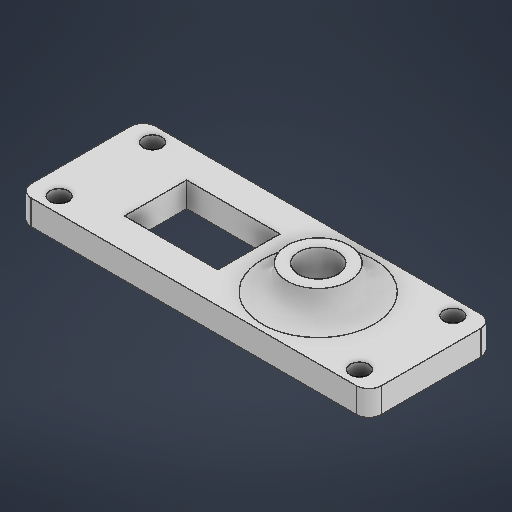
# Autodesk Inventor part: back_servo_support
Saved by Autodesk Inventor 2026.1 (Build 301233000, 233)
## iProperties
Created: 2025-10-30
Part Number: back_servo_support
Material: Generic
Document SubType Name: Modeling
Designer: emanuel
Density: 1 g/cm^3
Appearance: Default
Author: emanuel
Autodesk Inventor part; units mm, degrees
ref_plane "YZ Plane" through (0, 0, 0) normal (1, 0, 0) x (0, 1, 0)
ref_plane "XZ Plane" through (0, 0, 0) normal (0, 1, 0) x (-1, 0, 0)
ref_plane "XY Plane" through (0, 0, 0) normal (0, 0, 1) x (1, 0, 0)
sketch "Sketch1" plane through (0, 0, 0) normal (0, 1, 0) x (-1, 0, 0)
  line L0 (0, 0) -> (48.3, 0)
  line L1 (48.3, 0) -> (48.3, -15)
  line L2 (48.3, -15) -> (0, -15)
  line L3 (0, -15) -> (0, 0)
  circle A0 centre (48.3, 0) radius 1.5
  circle A1 centre (48.3, -15) radius 1.5
  circle A2 centre (0, 0) radius 1.5
  circle A3 centre (0, -15) radius 1.5
  line L4 (48.3, -15) -> (52.3, -15)
  line L5 (52.3, -15) -> (52.3, -17.5)
  line L6 (52.3, -17.5) -> (48.3, -17.5)
  line L7 (48.3, -17.5) -> (48.3, -15)
  line L8 (0, 0) -> (-4, 0)
  line L9 (-4, 0) -> (-4, 2.5)
  line L10 (-4, 2.5) -> (0, 2.5)
  line L11 (0, 2.5) -> (0, 0)
  line L12 (-4, 2.5) -> (52.3, 2.5)
  line L13 (52.3, 2.5) -> (52.3, -17.5)
  line L14 (52.3, -17.5) -> (-4, -17.5)
  line L15 (-4, -17.5) -> (-4, 2.5)
  dimension "d0" = 48.3
  dimension "d1" = 15
  dimension "d2" = 3
  dimension "d3" = 3
  dimension "d4" = 3
  dimension "d5" = 3
  dimension "d6" = 4
  dimension "d7" = 2.5
  dimension "d8" = 4
  dimension "d9" = 2.5
  constraints: 32 end point, 8 parallel, 4 centre point, 4 coincident, 4 horizontal, 4 perpendicular
  measures "d0" distance of L1.end L2.end
  measures "d1" distance of L0.end L1.end
  measures "d2" diameter of A0
  measures "d3" diameter of A1
  measures "d4" diameter of A2
  measures "d5" diameter of A3
  measures "d6" distance of L5.end L6.end
  measures "d7" distance of L4.end L5.end
  measures "d8" distance of L9.end L10.end
  measures "d9" distance of L8.end L9.end
extrude "Extrusion1" add sketch "Sketch1" along normal blind 4 contours A2 L11 L12 L13 L4 A1 L1 A0 L0 | L0 A0 L1 A1 L2 A3 L3 A2 | L3 A3 L2 A1 L7 L14 L15 L8 A2 | L8 L9 L10 L11 A2 | L7 A1 L4 L5 L6
sketch "Sketch2" plane through (0, 4, 0) normal (0, 1, 0) x (1, 0, 0)
  line L0 (4, -2.5) -> (4, 17.5) projected
  line L1 (4, -2.5) -> (-14.15, -2.5)
  line L2 (-14.15, -2.5) -> (-14.15, 7.5)
  line L3 (-14.15, 7.5) -> (4, 7.5)
  line L4 (4, 7.5) -> (4, -2.5)
  circle A0 centre (-14.15, 7.5) radius 5
  circle A1 centre (-14.15, 7.5) radius 3.15
  point P0 (0, 0)
  dimension "d12" = 18.15
  dimension "d13" = 10
  dimension "d14" = 10
  dimension "d19" = 6.3
  constraints: 8 end point, 2 centre point, 2 parallel, 1 coincident, 1 horizontal, 1 perpendicular
  measures "d12" distance of L2.end L3.end
  measures "d13" distance of L1.end L2.end
  measures "d14" diameter of A0
  measures "d19" diameter of A1
extrude "Extrusion2" add sketch "Sketch2" along normal blind 4 contours A0 L2 A1 L3 | L3 A1 L2 A0
extrude "Extrusion3" cut sketch "Sketch2" against normal blind 3 contours A1 L2 L3 | L3 L2 A1
fillet "Fillet2" radius 4 1 edges at (-19.15, 4, -7.5)
sketch "Sketch3" plane through (0, 4, 0) normal (0, 1, 0) x (1, 0, 0)
  line L0 (4, 17.5) -> (-52.3, 17.5) projected
  line L1 (-52.3, 17.5) -> (-40.3, 17.5)
  line L2 (-40.3, 17.5) -> (-40.3, 12.5)
  line L3 (-40.3, 12.5) -> (-52.3, 12.5)
  line L4 (-52.3, 12.5) -> (-52.3, 17.5)
  line L5 (-52.3, -2.5) -> (4, -2.5) projected
  line L6 (-52.3, -2.5) -> (-40.3, -2.5)
  line L7 (-40.3, -2.5) -> (-40.3, 2.5)
  line L8 (-40.3, 2.5) -> (-52.3, 2.5)
  line L9 (-52.3, 2.5) -> (-52.3, -2.5)
  line L10 (-40.3, 2.5) -> (-25.3, 2.5)
  line L11 (-25.3, 2.5) -> (-25.3, 12.5)
  line L12 (-25.3, 12.5) -> (-40.3, 12.5)
  line L13 (-40.3, 12.5) -> (-40.3, 2.5)
  point P0 (0, 0)
  dimension "d25" = 12
  dimension "d26" = 5
  dimension "d27" = 12
  dimension "d28" = 5
  dimension "d29" = 15
  constraints: 24 end point, 6 parallel, 3 horizontal, 3 perpendicular, 1 point on line
  measures "d25" distance of L2.end L3.end
  measures "d26" distance of L1.end L2.end
  measures "d27" distance of L8.end L7.end
  measures "d28" distance of L7.end L6.end
  measures "d29" distance of L12.end L11.end
extrude "Extrusion4" cut sketch "Sketch3" against normal blind 4 contours L12 L11 L10 L13
fillet "Fillet3" radius 2 4 edges at (-52.3, 2, 2.5) (4, 2, 2.5) (4, 2, -17.5) (-52.3, 2, -17.5)
body "Solid1"
